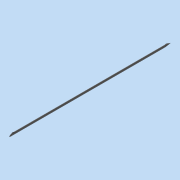
# Autodesk Inventor part: PrimaryHullWireCover
Saved by Autodesk Inventor 2017 (Build 210142000, 142)
## iProperties
Created: 2017-04-13
Part Number: PrimaryHullWireCover
Material: Carbon Fiber PLA
Document SubType Name: Modeling
Designer: Derek Wider
Mass: 12.8156 g
Surface Area: 126.956 cm^2
Volume: 9.85091 cm^3
Density: 1.30096 g/cm^3
Appearance: C-PLA Black
Author: Derek Wider
Autodesk Inventor part; units mm, degrees
ref_plane "YZ Plane" through (0, 0, 0) normal (1, 0, 0) x (0, 1, 0)
ref_plane "XZ Plane" through (0, 0, 0) normal (0, 1, 0) x (-1, 0, 0)
ref_plane "XY Plane" through (0, 0, 0) normal (0, 0, 1) x (1, 0, 0)
sketch "Sketch1" plane through (0, 0, 0) normal (0, 0, 1) x (1, 0, 0)
  arc A0 (10.7315, 12.5465) -> (0, 0) centre (12.7, 0) ccw
  arc A1 (10.7315, 12.5465) -> (0, 0) centre (43.4573, -26.3079) ccw
  dimension "d4" = 12.7
  dimension "d5" = 50.8
  dimension "d6" = 16.51
  constraints: 4 point on circle, 2 centre point, 1 coincident, 1 horizontal alignment, 1 other
  measures "d4" radius of A0
  measures "d5" radius of A1
  measures "d6" distance of point (0, 0) A0.start
extrude "Extrusion1" add sketch "Sketch1" against normal blind 355.6
sketch "Sketch2" plane through (0, 0, 0) normal (0, 0, 1) x (1, 0, 0)
  arc A0 (10.7315, 12.5465) -> (0, 0) centre (12.7, 0) ccw projected
  arc A1 (10.7315, 12.5465) -> (0, 0) centre (43.4573, -26.3079) ccw projected
  line L0 (3.0488, 8.255) -> (4.8526, 6.7121)
  constraints: 2 end point, 2 point on circle
revolve "Revolution1" add sketch "Sketch2" angle 180 about axis through (3.0488, 8.255, 0) along (0.7599342, -0.65, 0) picked at (4.3822, 8.4163) contours A1 L0 A0
sketch "Sketch4" plane through (0, 0, -355.6) normal (0, 0, -1) x (-1, 0, 0)
  arc A0 (0, 0) -> (-10.7315, 12.5465) centre (-12.7, 0) ccw projected
  arc A1 (0, 0) -> (-10.7315, 12.5465) centre (-43.4573, -26.3079) ccw projected
  line L0 (-3.0488, 8.255) -> (-4.8526, 6.7121)
  constraints: 2 end point, 2 point on circle
revolve "Revolution2" add sketch "Sketch4" angle 180 about axis through (3.0488, 8.255, -355.6) along (0.7599342, -0.65, 0) picked at (-3.0961, 6.9127) contours A1 L0 A0
sketch "Sketch5" plane through (0, 0, 0) normal (0, 0, 1) x (1, 0, 0)
  arc A0 (10.7315, 12.5465) -> (0, 0) centre (43.4573, -26.3079) ccw projected
  line L0 (0, 0) -> (10.7315, 12.5465) projected
extrude "Extrusion2" cut sketch "Sketch5" along normal through all both and the other way through all
body "Solid1"
